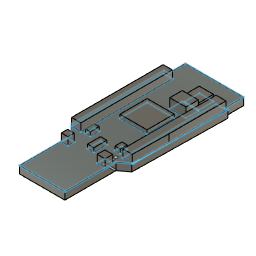
TSDZ2 remote box - garmin mount v47 (Autodesk Fusion 360 archive; units mm, degrees)
design "nrf52"
Autodesk Fusion 360 part; units mm, degrees
sketch "Sketch1" plane through (0, 0, 0) normal (0, 0, 1) x (1, 0, 0)
  line L0 (7.0671, 47.8249) -> (22.3102, 47.8249)
  line L1 (22.3102, 47.8249) -> (22.3102, 42.9285)
  line L2 (22.3102, 42.9285) -> (23.1024, 42.9285)
  line L3 (23.1024, 42.9285) -> (22.7044, 18.166)
  line L4 (22.7044, 18.166) -> (20.3351, 16.3902)
  line L5 (20.3351, 16.3902) -> (20.3351, 3.0086)
  line L6 (20.3351, 3.0086) -> (8.4669, 3.0086)
  line L7 (8.4669, 3.0086) -> (8.4669, 16.5034)
  line L8 (8.4669, 16.5034) -> (5.8161, 19.3048)
  line L9 (5.8161, 19.3048) -> (5.8161, 43.4328)
  line L10 (5.8161, 43.4328) -> (7.0671, 43.4328)
  line L11 (7.0671, 43.4328) -> (7.0671, 47.8249)
  line L12 (15.2672, 35.5395) -> (15.2672, 38.7967)
  line L13 (15.2672, 38.7967) -> (19.5064, 38.7967)
  line L14 (19.5064, 38.7967) -> (19.5064, 35.5395)
  line L15 (19.5064, 35.5395) -> (15.2672, 35.5395)
  line L16 (15.6085, 39.0819) -> (15.6085, 42.9261)
  line L17 (15.6085, 42.9261) -> (19.3493, 42.9261)
  line L18 (19.3493, 42.9261) -> (19.3493, 39.0523)
  line L19 (19.3493, 39.0523) -> (15.6085, 39.0819)
  line L20 (10.8921, 34.0033) -> (17.9754, 34.0033)
  line L21 (17.9754, 34.0033) -> (17.9754, 26.8691)
  line L22 (17.9754, 26.8691) -> (10.8921, 26.8691)
  line L23 (10.8921, 26.8691) -> (10.8921, 34.0033)
  line L24 (13.5241, 19.1586) -> (15.1785, 19.1586)
  line L25 (15.1785, 19.1586) -> (15.1785, 15.7525)
  line L26 (15.1785, 15.7525) -> (13.5241, 15.7525)
  line L27 (13.5241, 15.7525) -> (13.5241, 19.1586)
  line L28 (9.826, 21.251) -> (11.0911, 21.251)
  line L29 (11.0911, 21.251) -> (11.0911, 18.9153)
  line L30 (11.0911, 18.9153) -> (9.826, 18.9153)
  line L31 (9.826, 18.9153) -> (9.826, 21.251)
  line L32 (17.5628, 20.7644) -> (18.9253, 20.7644)
  line L33 (18.9253, 20.7644) -> (18.9253, 18.9153)
  line L34 (18.9253, 18.9153) -> (17.5628, 18.9153)
  line L35 (17.5628, 18.9153) -> (17.5628, 20.7644)
  line L36 (6.3955, 42.6771) -> (8.838, 42.6771)
  line L37 (8.838, 42.6771) -> (8.838, 18.6925)
  line L38 (8.838, 18.6925) -> (6.3955, 18.6925)
  line L39 (6.3955, 18.6925) -> (6.3955, 42.6771)
  line L40 (20.2451, 42.6771) -> (22.8585, 42.6771)
  line L41 (22.8585, 42.6771) -> (22.8585, 18.2815)
  line L42 (22.8585, 18.2815) -> (20.2451, 18.2815)
  line L43 (20.2451, 18.2815) -> (20.2451, 42.6771)
  line L44 (8.5715, 15.5042) -> (10.3004, 15.5042)
  line L45 (10.3004, 15.5042) -> (10.3004, 13.8543)
  line L46 (10.3004, 13.8543) -> (8.5715, 13.8543)
  line L47 (8.5715, 13.8543) -> (8.5715, 15.5042)
  line L48 (20.15, 15.7215) -> (18.1149, 15.7215)
  line L49 (18.1149, 15.7215) -> (18.1149, 13.7259)
  line L50 (18.1149, 13.7259) -> (20.15, 13.7259)
  line L51 (20.15, 13.7259) -> (20.15, 15.7215)
  constraint horizontal L0
  constraint perpendicular L0 L1
  constraint perpendicular L1 L2
  constraint vertical L5
  constraint perpendicular L5 L6
  constraint perpendicular L6 L7
  constraint perpendicular L6 L9
  constraint perpendicular L9 L10
  constraint perpendicular L0 L11
  constraint vertical L12
  constraint perpendicular L12 L13
  constraint perpendicular L13 L14
  constraint perpendicular L12 L15
  constraint perpendicular L13 L16
  constraint perpendicular L16 L17
  constraint perpendicular L13 L18
  constraint horizontal L20
  constraint vertical L21
  constraint horizontal L22
  constraint vertical L23
  constraint horizontal L24
  constraint vertical L25
  constraint horizontal L26
  constraint vertical L27
  constraint horizontal L28
  constraint vertical L29
  constraint horizontal L30
  constraint vertical L31
  constraint horizontal L32
  constraint vertical L33
  constraint horizontal L34
  constraint vertical L35
  constraint horizontal L36
  constraint vertical L37
  constraint horizontal L38
  constraint vertical L39
  constraint horizontal L40
  constraint vertical L41
  constraint horizontal L42
  constraint vertical L43
  constraint coincident L4 L41.end
  constraint horizontal L44
  constraint vertical L45
  constraint horizontal L46
  constraint vertical L47
  constraint horizontal L48
  constraint vertical L49
  constraint horizontal L50
  constraint vertical L51
extrude "Extrude13" add sketch "Sketch1" along normal blind 2 contours L44 L45 L46 L47 | L48 L49 L50 L51 makes body 1 at (9.1478, 15.5042, 0.6667) makes body 2 at (18.7933, 13.7259, 0.6667)
extrude "Extrude12" add sketch "Sketch1" along normal blind 2 separate body contours L36 L37 L38 L39 | L3 L40 L41 L42 L43 makes body 3 at (7.2097, 34.6822, 0) makes body 4 at (21.1163, 29.5705, 0)
extrude "Extrude11" add sketch "Sketch1" along normal blind 1 separate body contours L28 L29 L30 L31 | L32 L33 L34 L35 makes body 5 at (10.6694, 19.6939, 0) makes body 6 at (18.017, 20.148, 0)
extrude "Extrude10" add sketch "Sketch1" along normal blind 1 separate body contours L24 L25 L26 L27 makes body 7
extrude "Extrude9" add sketch "Sketch1" along normal blind 0.9 separate body contours L20 L21 L22 L23 makes body 8
extrude "Extrude6" add sketch "Sketch1" along normal blind 1.6 separate body contours L16 L17 L18 L19 makes body 9
extrude "Extrude7" add sketch "Sketch1" along normal blind 2.5 separate body contours L12 L13 L14 L15 makes body 10
extrude "Extrude8" add sketch "Sketch1" against normal blind 1.92 separate body contours L36 L37 L38 L39 | L0 L1 L2 L3 L4 L5 L6 L7 L8 L9 L10 L11 L40 L41 L42 L43 | L3 L40 L41 L42 L43 | L20 L21 L22 L23 | L24 L25 L26 L27 | L28 L29 L30 L31 | L32 L33 L34 L35 | L44 L45 L46 L47 | L48 L49 L50 L51 makes body 11
